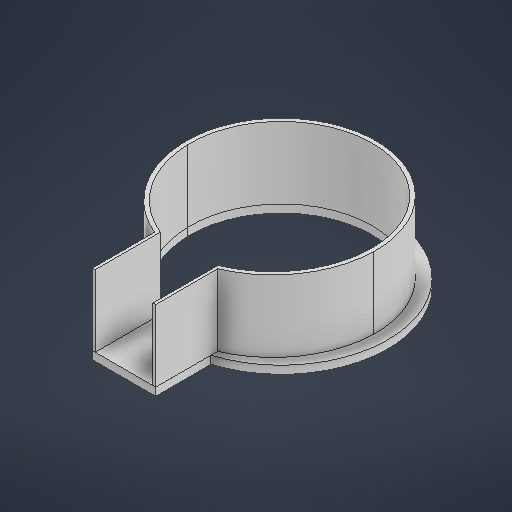
# Autodesk Inventor part: Cylinder Housing Optical Camera
Saved by Autodesk Inventor 2025 (Build 290162000, 162)
## iProperties
Created: 2025-08-14
Part Number: Cylinder Housing Optical Camera
Material: Generic
Document SubType Name: Modeling
Designer: mayhem
Density: 1 g/cm^3
Appearance: Default
Author: mayhem
Autodesk Inventor part; units mm, degrees
ref_plane "YZ Plane" through (0, 0, 0) normal (1, 0, 0) x (0, 1, 0)
ref_plane "XZ Plane" through (0, 0, 0) normal (0, 1, 0) x (-1, 0, 0)
ref_plane "XY Plane" through (0, 0, 0) normal (0, 0, 1) x (1, 0, 0)
sketch "Sketch1" plane through (0, 0, 0) normal (0, 1, 0) x (-1, 0, 0)
  arc A0 (-40.0043, 128.9366) -> (39.9957, 128.9393) centre (0, 0) ccw
  line L0 (-40.0043, 128.9366) -> (-40.0043, 198.9366)
  line L1 (-40.0043, 198.9366) -> (39.9957, 198.9366)
  line L2 (39.9957, 198.9366) -> (39.9957, 128.9393)
  arc A1 (-114.9519, 3.3257) -> (114.9519, 3.3257) centre (0, 0) ccw
  arc A2 (114.9519, 3.3257) -> (39.9957, 115.0039) centre (-11.1576, -0.3228) ccw
  line L3 (0, -135) -> (0, -115)
  arc A3 (-39.9957, 115.0039) -> (-114.9519, 3.3257) centre (11.1576, -0.3228) ccw
  arc A4 (39.9957, 115.0039) -> (-39.9957, 115.0039) centre (0, 24.8323) ccw
  point P0 (0, 128.7652)
  point P1 (-0.0043, -3.5634)
  point P2 (-0.0043, 198.9366)
  dimension "d0" = 270
  dimension "d7" = 80
  dimension "d9" = 230
  dimension "d13" = 70
  constraints: 14 point on circle, 8 end point, 5 centre point, 3 tangent, 2 coincident, 2 symmetric about line, 1 midpoint, 1 parallel, 1 vertical, 1 other
  measures "d0" diameter of A0
  measures "d7" distance of L0.end L1.end
  measures "d9" diameter of A1
  measures "d13" distance of L0.start L0.end
extrude "Extrusion1" add sketch "Sketch1" along normal blind 10
sketch "Sketch2" plane through (0, 10, 0) normal (0, 1, 0) x (-1, 0, 0.000033)
  arc A0 (-114.954, 3.2517) -> (114.954, 3.2517) centre (0, 0) ccw
  arc A1 (-40, 128.938) -> (40, 128.938) centre (0, 0) ccw projected
  arc A2 (114.954, 3.2517) -> (39.9995, 115.0026) centre (-10.9119, -0.1577) ccw
  arc A3 (-39.9919, 115.0052) -> (-114.954, 3.2517) centre (11.1458, -0.3153) ccw
  arc A4 (-119.952, 3.3931) -> (119.9521, 3.3901) centre (0, 0) ccw
  arc A5 (119.9521, 3.3901) -> (40.0023, 120.448) centre (-10.9119, -0.1577) ccw
  arc A6 (-39.9977, 120.452) -> (-119.952, 3.3931) centre (11.1458, -0.3153) ccw
  line L0 (-39.9977, 198.938) -> (-39.9977, 120.4492)
  line L1 (39.9944, 115.0072) -> (40.0032, 115.0072)
  line L2 (40.0023, 120.4456) -> (40.0023, 198.9353)
  line L3 (-36.4977, 116.4776) -> (-36.4977, 198.938)
  line L4 (36.5031, 198.9353) -> (36.5031, 116.4761)
  arc A7 (114.9561, 3.2518) -> (39.9998, 115.0048) centre (-10.9119, -0.1577) ccw
  arc A8 (-114.9561, 3.2518) -> (114.9561, 3.2518) centre (0, 0) ccw
  arc A9 (-39.9681, 115.0181) -> (-114.9561, 3.2518) centre (11.1458, -0.3153) ccw
  arc A10 (39.9998, 115.0048) -> (36.5031, 116.4761) centre (0.0008, 24.8323) ccw
  arc A11 (-36.4977, 116.4776) -> (-39.9681, 115.0181) centre (0.0008, 24.8323) ccw
  line L5 (40.0023, 198.9353) -> (36.5031, 198.9353)
  line L6 (-36.4977, 198.938) -> (-39.9977, 198.938)
  point P0 (39.9995, 115.0026)
  point P1 (-39.9919, 115.0052)
  dimension "d15" = 5
  dimension "d16" = 3.5
  constraints: 23 point on circle, 14 end point, 11 centre point, 4 parallel, 3 coincident, 2 horizontal, 2 perpendicular, 2 point on line, 1 tangent
  measures "d15" radial gap between concentric circles of A3 A6
  measures "d16" distance between parallel lines of L0 L3
extrude "Extrusion2" add sketch "Sketch2" along normal blind 90.5
body "Solid1"
